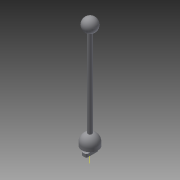
# Autodesk Inventor part: EarShapeET
Saved by Autodesk Inventor 2014 SP1 (Build 180222100, 222)
## iProperties
Created: 2013-10-30
Part Number: EarShapeET
Material: Generic
Document SubType Name: Modeling
Designer: david
Density: 1 g/cm^3
Appearance: Default
Mass: 53.4443 g
Surface Area: 145.67 cm^2
Volume: 53.4443 cm^3
Author: david
Autodesk Inventor part; units mm, degrees
ref_plane "YZ Plane" through (0, 0, 0) normal (1, 0, 0) x (0, 1, 0)
ref_plane "XZ Plane" through (0, 0, 0) normal (0, 1, 0) x (-1, 0, 0)
ref_plane "XY Plane" through (0, 0, 0) normal (0, 0, 1) x (1, 0, 0)
sketch "Sketch1" plane through (0, 0, 0) normal (0, 1, 0) x (-1, 0, 0)
  circle A0 centre (0, 0) radius 7.5
  dimension "d0" = 15
  constraints: 1 centre point, 1 coincident
  measures "d0" diameter of A0
extrude "Extrusion1" add sketch "Sketch1" along normal blind 3
sketch "Sketch2" plane through (0, 0, 0) normal (0, -1, 0) x (1, 0, 0)
  circle A0 centre (0, 0) radius 7.5 projected
  circle A1 centre (0, 0) radius 2.3
  dimension "d3" = 4.6
  constraints: 1 centre point, 1 coincident
  measures "d3" diameter of A1
extrude "Extrusion2" add sketch "Sketch2" along normal blind 3.2 contours A1
sketch "Sketch3" plane through (0, -3.2, 0) normal (0, -1, 0) x (1, 0, 0)
  circle A0 centre (0, 0) radius 2.3 projected
  line L0 (-2.3, 5.3245) -> (-2.3, -5.3245)
  line L1 (2.3, 5.3245) -> (2.3, -5.3245)
  line L2 (0, 15.7328) -> (0, -15.032) construction
  circle A1 centre (0, 0) radius 7.5 construction
  arc A2 (-3, 6.8739) -> (-3, -6.8739) centre (0, 0) ccw construction
  arc A3 (3, -6.8739) -> (3, 6.8739) centre (0, 0) ccw construction
  arc A4 (2.3, 5.3245) -> (-2.3, 5.3245) centre (0, 0) ccw
  arc A5 (-2.3, -5.3245) -> (2.3, -5.3245) centre (0, 0) ccw
  dimension "d13" = 5.8
  dimension "d19" = 5.8
  constraints: 12 point on circle, 6 end point, 4 centre point, 2 coincident, 2 parallel, 2 tangent, 1 concentric, 1 vertical
  measures "d13" radius of A4
  measures "d19" radius of A5
extrude "Extrusion3" add sketch "Sketch3" along normal blind 2.8
fillet "Fillet2" radius 1.2 4 edges at (-2.3, -4.6, 5.3245) (2.3, -4.6, 5.3245) (-2.3, -4.6, -5.3245) (2.3, -4.6, -5.3245)
ref_plane "Work Plane1" through (0, -3.2, 2.3) normal (1, 0, 0) x (0, 0, -1)
sketch "Sketch8" plane through (0, -3.2, 2.3) normal (1, 0, 0) x (0, 0, -1)
  line L0 (-3.5, -2.8) -> (26.5, -2.8) construction
  line L1 (-63.9924, 6.2) -> (53.0342, 6.2) construction
  line L2 (9.8, 3.2) -> (9.8, -146.8) construction
  arc A0 (9.8, 6.2) -> (4.3, 13.4284) centre (2.3, 6.2) ccw
  line L3 (-3.5, -2.8) -> (-3.0245, -2.8) projected
  line L4 (4.3, 13.4284) -> (4.3, 6.2)
  line L5 (4.3, 6.2) -> (9.8, 6.2)
  line L6 (-5.2, 3.2) -> (9.8, 3.2) projected
  line L7 (2.3, 3.2) -> (9.8, 3.2) construction
  line L8 (2.3, 6.2) -> (4.3, 6.2)
  line L9 (4.3, 6.2) -> (4.3, 105.8714)
  line L10 (2.3, 106.2) -> (2.3, 6.2)
  line L11 (2.3, 3.2) -> (2.3, 202.2325) construction
  arc A1 (2.3, 93.7) -> (2.3, 106.2) centre (2.3, 99.95) ccw
  line L12 (2.3, 106.2) -> (2.3, 93.7) construction
  line L13 (4.3, 105.8714) -> (2.3, 106.2)
  line L14 (2.3, 106.2) -> (2.3, 93.7)
  line L15 (2.3, -217.6065) -> (2.3, 271.0391) projected
  point P0 (37.0288, 0)
  point P1 (-3.3317, -2.8)
  dimension "d54" = 30
  dimension "d58" = 9
  dimension "d61" = 150
  dimension "d64" = 0
  dimension "d65" = 2
  dimension "d66" = 100
  dimension "d68" = 7.5
  dimension "d70" = 6.25
  constraints: 26 end point, 6 collinear, 6 point on line, 5 point on circle, 2 centre point, 2 horizontal, 2 parallel, 1 perpendicular
  measures "d54" distance of L0.start L0.end
  measures "d58" distance between parallel lines of L0 L1
  measures "d61" distance of L2.start L2.end
  measures "d64" distance from line of L3 L0.start
  measures "d65" distance between parallel lines of L9 L10
  measures "d66" distance of L10.start L8.start
  measures "d68" radius of A0
  measures "d70" radius of A1
revolve "Revolution4" add sketch "Sketch8" angle 360 about axis through (0, 3, 0) along (0, 1, 0)
equation "\"d0\" = HeadConnectorOuterSize"
equation "\"d1\" = EarConnectorHeight"
equation "\"d3\" = HeadConnectorWidth - HeadConnectorTolerance"
equation "\"d4\" = HeadConnectorOuterHeight + HeadConnectorTolerance"
equation "\"d13\" = 0.5 * HeadConnectorDiam - HeadConnectorTolerance"
equation "\"d19\" = 0.5 * HeadConnectorDiam - HeadConnectorTolerance"
equation "\"d10\" = HeadConnectorHeight - HeadConnectorTolerance"
equation "\"d20\" = 2 * HeadConnectorProportion"
equation "\"d58\" = HeadConnectorOuterHeight + HeadConnectorHeight + EarConnectorHeight"
equation "\"d65\" = 0.5 * EarWidth"
equation "\"d66\" = EarHeight"
equation "\"d68\" = 0.5 * HeadConnectorOuterSize"
equation "\"d70\" = 0.5 * EarBallSize"
equation "\"EarHeight\" = 100"
equation "\"EarWidth\" = 4"
equation "\"EarBallSize\" = 12.5"
equation "\"HeadConnectorOuterSize\" = 15"
equation "\"EarConnectorHeight\" = 3"
equation "\"HeadConnectorWidth\" = 4.8"
equation "\"HeadConnectorTolerance\" = 0.2"
equation "\"HeadConnectorOuterHeight\" = 3"
equation "\"HeadConnectorDiam\" = 12"
equation "\"HeadConnectorHeight\" = 3"
equation "\"HeadConnectorProportion\" = 0.6"
body "Solid1"
